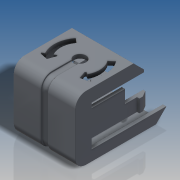
# Autodesk Inventor part: 99397-LtBluishGray
Saved by Autodesk Inventor 2016 SP2 (Build 200236200, 236)
## iProperties
Created: 2015-08-28
Part Number: 99397-LtBluishGray
Material: ABS Plastic
Document SubType Name: Modeling
Designer: D. Kohfeld
Density: 1.06 g/cm^3
Appearance: LtBluishGray
Mass: 2.55562 g
Surface Area: 41.4756 cm^2
Volume: 2.41097 cm^3
Author: D. Kohfeld
Autodesk Inventor part; units mm, degrees
ref_plane "YZ Plane" through (0, 0, 0) normal (1, 0, 0) x (0, 1, 0)
ref_plane "XZ Plane" through (0, 0, 0) normal (0, 1, 0) x (-1, 0, 0)
ref_plane "XY Plane" through (0, 0, 0) normal (0, 0, 1) x (1, 0, 0)
sketch "Sketch2" plane through (0, 0, 0) normal (1, 0, 0) x (0, 1, 0)
  line L0 (-10.8, -21.6) -> (-10.8, 2)
  arc A0 (-7.2, 5.6) -> (-10.8, 2) centre (-7.2, 2) ccw
  line L1 (-7.2, 5.6) -> (7.2, 5.6)
  arc A1 (10.8, 2) -> (7.2, 5.6) centre (7.2, 2) ccw
  line L2 (10.8, 2) -> (10.8, -14)
  line L3 (10.8, -14) -> (7.2, -17.6)
  line L4 (7.2, -17.6) -> (6.4, -17.6)
  line L5 (6.4, -17.6) -> (6.4, 0)
  line L6 (6.4, 0) -> (4.8, 0)
  line L7 (4.8, 0) -> (4.8, -11.2)
  line L8 (4.8, -11.2) -> (0.4, -11.2)
  line L9 (0.4, -11.2) -> (0.4, -15.2)
  line L10 (0.4, -15.2) -> (-4, -15.2)
  line L11 (-4, -15.2) -> (-4, 0)
  line L12 (-4, 0) -> (-7.2, 0)
  line L13 (-7.2, 0) -> (-7.2, -25.2)
  line L14 (-7.2, -25.2) -> (-10.8, -21.6)
  line L15 (9.36, -15.44) -> (9.36, 4)
  line L16 (9.36, 4) -> (-9.6, 4)
  line L17 (-9.6, 4) -> (-9.6, -22.8)
  line L18 (-9.6, 3.2) -> (9.36, 3.2)
  line L19 (10.8, -6.4) -> (10.4, -6.4)
  line L20 (10.4, -6.4) -> (10.4, 2)
  arc A2 (10.4, 2) -> (7.2, 5.2) centre (7.2, 2) ccw
  line L21 (7.2, 5.2) -> (-7.2, 5.2)
  arc A3 (-7.2, 5.2) -> (-10.4, 2) centre (-7.2, 2) ccw
  line L22 (-10.4, 2) -> (-10.4, -6.8)
  line L23 (-10.4, -6.8) -> (-10.8, -6.8)
  line L24 (-10.8, -10.8) -> (-9.6, -10.8)
  point P0 (0, 0)
  point P1 (0, 5.6)
  dimension "d0" = 21.6
  dimension "d1" = 3.6
  dimension "d2" = 30.8
  dimension "d3" = 5.6
  dimension "d4" = 45
  dimension "d5" = 3.6
  dimension "d6" = 4.4
  dimension "d7" = 4.4
  dimension "d8" = 4.4
  dimension "d9" = 0.8
  dimension "d10" = 23.2
  dimension "d11" = 1.6
  dimension "d12" = 16.8
  dimension "d13" = 20.8
  dimension "d14" = 1.44
  dimension "d15" = 1.2
  dimension "d16" = 1.6
  dimension "d17" = 0.8
  dimension "d18" = 0.4
  dimension "d19" = 12
  dimension "d20" = 12.4
  dimension "d21" = 14.4
  constraints: 50 end point, 12 horizontal, 11 vertical, 8 point on circle, 8 point on line, 8 tangent, 4 centre point, 2 concentric, 2 horizontal alignment, 1 equal radius, 1 midpoint, 1 perpendicular, 1 vertical alignment
  measures "d0" distance between parallel lines of L2 L0
  measures "d1" radius of A1
  measures "d2" distance from line of L13.end L1
  measures "d3" distance between parallel lines of L12 L1
  measures "d4" angle of L13 L14
  measures "d5" distance between parallel lines of L0 L13
  measures "d6" distance between parallel lines of L7 L9
  measures "d7" distance between parallel lines of L11 L9
  measures "d8" distance between parallel lines of L5 L2
  measures "d9" distance of L3.end L4.end
  measures "d10" distance from line of L3.end L1
  measures "d11" distance between parallel lines of L5 L7
  measures "d12" distance between parallel lines of L8 L1
  measures "d13" distance between parallel lines of L10 L1
  measures "d14" distance between parallel lines of L2 L15
  measures "d15" distance between parallel lines of L0 L17
  measures "d16" distance between parallel lines of L1 L16
  measures "d17" distance between parallel lines of L16 L18
  measures "d18" distance between parallel lines of L1 L21
  measures "d19" distance from line of L19.start L1
  measures "d20" distance from line of L23.end L1
  measures "d21" distance from line of L13.end L24
extrude "Extrusion1" add sketch "Sketch2" along normal mid plane 20.8
extrude "Extrusion2" cut sketch "Sketch2" along normal mid plane 18.4 contours L17 L18 L15 L3 L4 L5 L6 L7 L8 L9 L10 L11 L12 L13 L14 | L17 L16 L15 L18
extrude "Extrusion3" add sketch "Sketch2" along normal mid plane 4 contours L17 L16 L15 L18
extrude "Extrusion4" cut sketch "Sketch2" along normal mid plane 2.222 contours L0 A0 L1 A1 L2 L19 L20 A2 L21 A3 L22 L23
extrude "Extrusion5" cut sketch "Sketch2" along normal mid plane 8 contours L0 L24 L17 L14
sketch "Sketch3" plane through (10.4, 0.4, -11.2) normal (0, 1, 0) x (1, 0, 0)
  line L0 (-1.2, 4) -> (0, 4) projected
  line L1 (-19.6, 0) -> (-19.6, 4) projected
  line L2 (-20.8, 4) -> (-19.6, 4) projected
  line L3 (-20.8, 0) -> (-20.8, 4) projected
  line L4 (-20.8, 0) -> (-19.6, 0) projected
  line L5 (-1.2, 4) -> (-1.2, 7.2)
  line L6 (-1.2, 7.2) -> (-0.4, 7.2)
  line L7 (-0.4, 7.2) -> (0.8, 5.2)
  line L8 (0.8, 4) -> (0, 4)
  line L9 (-19.6, 4) -> (-19.6, 7.2)
  line L10 (-19.6, 7.2) -> (-20.4, 7.2)
  line L11 (-20.4, 7.2) -> (-21.6, 5.2)
  line L12 (-21.6, 4) -> (-20.8, 4)
  line L13 (0.8, 5.2) -> (0.8, 4)
  line L14 (-21.6, 5.2) -> (-21.6, 4)
  point P0 (-10.4, -11.2)
  dimension "d32" = 3.2
  dimension "d33" = 0.8
  dimension "d34" = 1.2
  dimension "d35" = 0.8
  constraints: 20 end point, 4 equal length, 4 horizontal, 4 vertical
  measures "d32" distance between parallel lines of L12 L10
  measures "d33" distance of L12.start L2.start
  measures "d34" distance of L11.end L12.start
  measures "d35" distance of L9.end L10.end
extrude "Extrusion6" add sketch "Sketch3" against normal up to surface (4.4 mm away) contours L5 L6 L7 L13 L8 L0 | L2 L12 L14 L11 L10 L9
sketch "Sketch4" plane through (-10.4, 10.8, -14) normal (0, 1, 0) x (1, 0, 0)
  line L0 (20.8, 0) -> (0, 0) projected
  line L1 (9.289, -7.6) -> (11.511, -7.6) projected
  circle A0 centre (10.4, -7.6) radius 2
  arc A1 (5.164, -3.582) -> (4.6557, -10.85) centre (10.4, -7.6) ccw
  arc A2 (3.6233, -2.3051) -> (2.9149, -11.8348) centre (10.4, -7.6) ccw
  line L2 (3.6233, -2.3051) -> (5.164, -3.582)
  line L3 (4.6557, -10.85) -> (5.4942, -10.3755)
  line L4 (5.4942, -10.3755) -> (5.7125, -10.7613)
  line L5 (2.9149, -11.8348) -> (2.0764, -12.3093)
  line L6 (2.0764, -12.3093) -> (2.2946, -12.695)
  line L7 (2.2946, -12.695) -> (4.8396, -13.2059)
  line L8 (4.8396, -13.2059) -> (5.7125, -10.7613)
  line L9 (10.4, -7.6) -> (10.4, -16)
  arc A3 (16.1443, -10.85) -> (15.636, -3.582) centre (10.4, -7.6) ccw
  arc A4 (17.8851, -11.8348) -> (17.1767, -2.3051) centre (10.4, -7.6) ccw
  line L10 (17.1767, -2.3051) -> (15.636, -3.582)
  line L11 (16.1443, -10.85) -> (15.3058, -10.3755)
  line L12 (15.3058, -10.3755) -> (15.0875, -10.7613)
  line L13 (17.8851, -11.8348) -> (18.7236, -12.3093)
  line L14 (18.7236, -12.3093) -> (18.5054, -12.695)
  line L15 (18.5054, -12.695) -> (15.9604, -13.2059)
  line L16 (15.9604, -13.2059) -> (15.0875, -10.7613)
  point P0 (9.289, -16)
  point P1 (10.4, -14)
  dimension "d38" = 4
  dimension "d39" = 39.65
  dimension "d40" = 8.6
  dimension "d41" = 6.6
  dimension "d42" = 98.3
  dimension "d43" = 3.927
  dimension "d44" = 2.141
  dimension "d45" = 69.15
  dimension "d46" = 5.236
  dimension "d47" = 4.018
  constraints: 30 end point, 9 symmetric about line, 8 point on circle, 5 centre point, 3 equal length, 2 coincident, 2 horizontal alignment, 2 point on line, 1 collinear, 1 midpoint, 1 parallel, 1 perpendicular, 1 vertical, 2 other
  measures "d38" diameter of A0
  measures "d39" angle of L0 L2
  measures "d40" radius of A2
  measures "d41" radius of A1
  measures "d42" angle of L8 L7
  measures "d43" distance between parallel lines of L4 L6
  measures "d44" distance from line of L7.end L3
  measures "d45" angle of L5 L2
  measures "d46" horizontal distance of A0.centre L2.end
  measures "d47" vertical distance of A0.centre L2.end
extrude "Extrusion7" cut sketch "Sketch4" against normal up to surface (1.44 mm away)
fillet "Fillet1" radius 0.1 159 edges at (-10.4, 10.8, -6) (-10.4, 0, 5.6) (-10.4, -9.7456, 4.5456) (-10.4, -10.8, -9.8) (-10.4, 9.7456, 4.5456) (10.4, 9.7456, 4.5456) (10.4, 0, 5.6) (10.4, -9.7456, 4.5456) (10.4, -10.8, -9.8) (10.4, 10.8, -6) (1.111, 9.7456, 4.5456) (1.111, 0, 5.6) (1.111, -9.7456, 4.5456) (1.111, -10.8, -2.4) (1.111, 10.8, -1.3685) (-1.111, 9.7456, 4.5456) (-1.111, 0, 5.6) (-1.111, -9.7456, 4.5456) (-1.111, -10.8, -2.4) (-1.111, 10.8, -1.3685) (6.5839, 10.8, -6.8605) (6.0064, 10.8, -11.0564) (8.5763, 10.8, -7.0375) (7.9044, 10.8, -1.9279) (7.4851, 10.08, -2.1652) (8.2145, 10.8, -1.4979) (6.8329, 10.8, -1.0496) (5.124, 10.8, -2.0164) (4.7966, 10.8, -3.4316) (5.3251, 10.8, -3.3872) (5.7443, 10.08, -3.15) (-0.9429, 10.8, -8.1638) (1.7638, 10.8, -5.4571) (0, 10.4, -4.4) (-2, 9.36, -6.4) (-1.111, 10.6, -4.737) (1.111, 10.6, -4.737) (-8.5763, 10.8, -7.0375) (-6.0064, 10.8, -11.0564) (-6.5839, 10.8, -6.8605) (-5.7443, 10.08, -3.15) (-5.3251, 10.8, -3.3872) (-4.7967, 10.8, -3.4316) (-5.124, 10.8, -2.0164) (-6.8329, 10.8, -1.0496) (-8.2145, 10.8, -1.4979) (-7.9044, 10.8, -1.9279) (-7.4851, 10.08, -2.1652) (-8.5763, 9.36, -7.0375) (-6.0064, 9.36, -11.0564) (-6.5839, 9.36, -6.8605) (-5.3251, 9.36, -3.3872) (-4.7967, 9.36, -3.4316) (-5.124, 9.36, -2.0164) (-6.8329, 9.36, -1.0496) (-8.2145, 9.36, -1.4979) (-7.9044, 9.36, -1.9279) (4.7966, 9.36, -3.4316) (5.3251, 9.36, -3.3872) (6.5839, 9.36, -6.8605) (5.124, 9.36, -2.0164) (6.8329, 9.36, -1.0496) (8.2145, 9.36, -1.4979) (7.9044, 9.36, -1.9279) (8.5763, 9.36, -7.0375) (6.0064, 9.36, -11.0564) (10.4, 6.4, -8.8) (10.4, 9, -15.8) (10.4, 6.8, -17.6) (10.4, 5.6, 0) (10.4, 4.8, -5.6) (10.4, 2.6, -11.2) (9.8, 4.8, -11.2) (9.2, 4.8, -5.6) (9.2, 5.6, 0) (9.2, 6.4, -8.8) (9.8, 6.4, -17.6) (9.8, 7.2, -17.6) (9.2, 6.8, -17.6) (9.2, 2.6, -11.2) (9.2, 0.4, -14.8) (10.4, 0.4, -13.2) (10.8, 0.4, -15.2) (11.2, -1.8, -15.2) (11.2, -1.8, -16.4) (11.2, 0.4, -15.8) (10.6, 0.4, -17.4) (9.6, 0.4, -18.4) (9.2, -1.8, -18.4) (10, -1.8, -18.4) (10.4, -4, -7.6) (10.8, -4, -15.2) (11.2, -4, -15.8) (10.6, -4, -17.4) (9.6, -4, -18.4) (9.2, -4, -9.2) (10.4, -5.6, 0) (9.2, -5.6, 0) (9.2, -7.2, -12.6) (10.4, -7.2, -12.6) (9.8, -7.2, -25.2) (10.4, -9, -23.4) (9.2, -8.4, -24) (6.6, -9.6, -22.8) (0, -9.6, -10.8) (-4, -9.6, -16.8) (-4, -10.8, -16.2) (0, -10.8, -10.8) (4, -9.6, -16.8) (4, -10.8, -16.2) (-4, -10.2, -22.2) (-6.6, -9.6, -22.8) (-9.2, -7.2, -12.6) (-10.4, -7.2, -12.6) (-9.2, -8.4, -24) (-9.8, -7.2, -25.2) (-10.4, -9, -23.4) (-9.2, -5.6, 0) (-10.4, -5.6, 0) (-9.2, -4, -9.2) (-10.4, -4, -7.6) (-11.2, -1.8, -15.2) (-10.8, -4, -15.2) (-11.2, -4, -15.8) (-10.6, -4, -17.4) (-9.2, -1.8, -18.4) (-9.6, -4, -18.4) (-10, -1.8, -18.4) (-9.6, 0.4, -18.4) (-10.6, 0.4, -17.4) (-11.2, -1.8, -16.4) (-11.2, 0.4, -15.8) (-10.4, 0.4, -13.2) (-9.2, 0.4, -14.8) (-9.2, 2.6, -11.2) (-10.4, 2.6, -11.2) (-9.8, 4.8, -11.2) (0, 9.36, -15.44) (0, 10.8, -14) (-9.2, 4.8, -5.6) (-10.4, 4.8, -5.6) (-9.2, 6.4, -8.8) (-9.2, 6.8, -17.6) (-9.8, 6.4, -17.6) (-10.4, 6.8, -17.6) (-9.8, 7.2, -17.6) (-9.2, 8.28, -16.52) (-10.4, 9, -15.8) (7.2, -10.8, -21.6) (4, -10.2, -22.2) (0, -10.8, -6.8) (-7.2, -10.8, -21.6) (2, -0.12, 3.2) (-2, -0.12, 3.2) (9.2, 8.28, -16.52) (-10.4, 5.6, 0) (-9.2, 5.6, 0) (-10.4, 6.4, -8.8) (-10.8, 0.4, -15.2)
equation "\"d11\" = wall"
equation "\"d16\" = wall"
equation "\"d30\" = lu"
equation "\"d36\" = lu"
equation "\"d48\" = lu"
equation "\"d50\" = lf"
equation "\"wall\" = 1.6"
equation "\"lu\" = 8"
equation "\"lf\" = 0.1"
body "Solid1"
